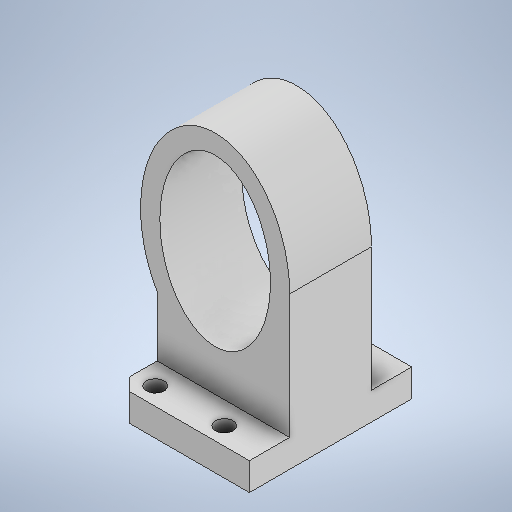
# Autodesk Inventor part: finger_hole_thumb
Saved by Autodesk Inventor 2025.2 (Build 292293000, 293)
## iProperties
Created: 2025-02-16
Part Number: finger_hole_thumb
Material: Generic
Document SubType Name: Modeling
Designer: Admin
Density: 1 g/cm^3
Appearance: Default
Author: Admin
Autodesk Inventor part; units mm, degrees
ref_plane "YZ Plane" through (0, 0, 0) normal (1, 0, 0) x (0, 1, 0)
ref_plane "XZ Plane" through (0, 0, 0) normal (0, 1, 0) x (-1, 0, 0)
ref_plane "XY Plane" through (0, 0, 0) normal (0, 0, 1) x (1, 0, 0)
sketch "Sketch1" plane through (0, 0, 0) normal (0, 1, 0) x (-1, 0, 0)
  circle A0 centre (7.962, -1.2776) radius 1.6
  circle A1 centre (-4.538, -1.2776) radius 1.6
  circle A2 centre (-4.538, 21.7224) radius 1.6
  circle A3 centre (7.962, 21.7224) radius 1.6
  line L0 (11.712, -2.1134) -> (11.712, 22.5582)
  line L1 (9.3478, -4.4776) -> (11.712, -2.1134)
  line L2 (-12.288, -4.4776) -> (9.3478, -4.4776)
  line L3 (-12.288, 24.9224) -> (-12.288, -4.4776)
  line L4 (9.3478, 24.9224) -> (-12.288, 24.9224)
  line L5 (11.712, 22.5582) -> (9.3478, 24.9224)
  point P0 (0, 0)
  dimension "d0" = 3.75
  dimension "d1" = 3.2
  dimension "d2" = 3.2
  dimension "d3" = 7.75
  dimension "d4" = 7.75
  dimension "d5" = 3.2
  dimension "d6" = 3.2
  dimension "d7" = 3.75
  dimension "d8" = 3.2
  dimension "d9" = 3.2
  dimension "d10" = 3.2
  dimension "d11" = 3.2
  constraints: 12 end point, 4 centre point
  measures "d0" distance from line of L0 A3.centre
  measures "d1" distance from line of L4 A3.centre
  measures "d2" distance from line of L4 A2.centre
  measures "d3" distance from line of L3 A2.centre
  measures "d4" distance from line of L3 A1.centre
  measures "d5" distance from line of L2 A1.centre
  measures "d6" distance from line of L2 A0.centre
  measures "d7" distance from line of L0 A0.centre
  measures "d8" diameter of A0
  measures "d9" diameter of A3
  measures "d10" diameter of A2
  measures "d11" diameter of A1
extrude "Extrusion1" add sketch "Sketch1" along normal blind 5
sketch "Sketch2" plane through (0, 5, 0) normal (0, 1, 0) x (1, 0, 0)
  line L0 (12.288, -24.9224) -> (12.288, 4.4776) projected
  line L1 (-11.712, -17.6224) -> (12.288, -17.6224)
  line L2 (12.288, -17.6224) -> (12.288, -2.8224)
  line L3 (12.288, -2.8224) -> (-11.712, -2.8224)
  line L4 (-11.712, -2.8224) -> (-11.712, -17.6224)
  circle A0 centre (-7.962, -21.7224) radius 1.6 projected
  circle A1 centre (-7.962, 1.2776) radius 1.6 projected
  line L5 (-11.712, 2.1134) -> (-11.712, -22.5582) projected
  point P0 (0, 0)
  point P1 (-11.712, -10.2224)
  dimension "d14" = 2.5
  dimension "d15" = 2.5
  dimension "d16" = 0
  constraints: 8 end point, 2 parallel, 1 horizontal, 1 midpoint, 1 perpendicular, 1 point on line
  measures "d14" distance edge to line of A0 L1
  measures "d15" distance edge to line of A1 L3
  measures "d16" distance from line of point (-11.712, -10.222) L4
extrude "Extrusion2" add sketch "Sketch2" along normal blind 4 contours L1 L4 L3 L0
sketch "Sketch3" plane through (-11.712, 5, 17.6224) normal (0, 0, 1) x (1, 0, 0)
  ellipse E0 centre (10.5, 22.5) end of major axis (10.5, 7.5) minor radius 10
  ellipse E1 centre (10.5, 22.5) end of major axis (10.5, 4) minor radius 13.5
  line L0 (0, 4) -> (24, 4) projected
  line L1 (24, 4) -> (24, 22.5)
  line L2 (24, 4) -> (10.5, 4)
  line L3 (0, 4) -> (0, 10.872)
  point P0 (11.712, -5)
  dimension "d21" = 13.5
  dimension "d22" = 18.5
  dimension "d19" = 10
  dimension "d20" = 15
  dimension "d23" = 18.5
  constraints: 6 end point, 3 vertical, 1 centre point, 1 coincident, 1 horizontal, 1 point on line, 6 other
  measures "d23" distance of L0.end L1.end
extrude "Extrusion3" add sketch "Sketch3" against normal blind 14.8
body "Solid1"
